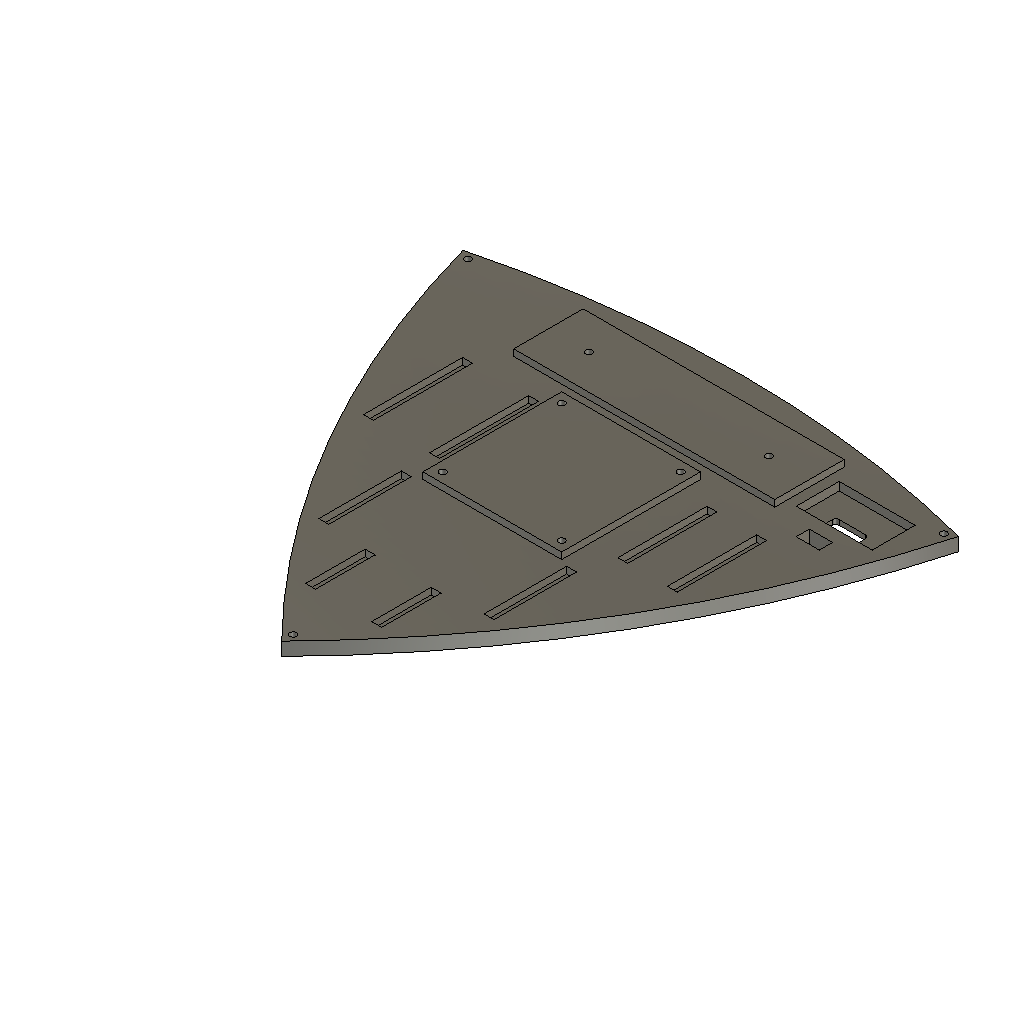
Body (Autodesk Fusion 360 design; units mm, degrees)
Autodesk Fusion 360 part; units mm, degrees
sketch "Base" plane through (0, 0, 0) normal (0, 0, 1) x (1, 0, 0)
  line L0 (0, 0) -> (150, 0)
  line L1 (150, 0) -> (75, -129.9038)
  line L2 (75, -129.9038) -> (0, 0)
  arc A0 (150, 0) -> (0, 0) centre (75, -290.4738) ccw
  arc A1 (0, 0) -> (75, -129.9038) centre (289.0576, 80.285) ccw
  arc A2 (75, -129.9038) -> (150, 0) centre (-139.0576, 80.285) ccw
  dimension "d1" = 150
  dimension "d2" = 150
  dimension "d3" = 150
  dimension "d4" = 300
  dimension "d5" = 300
  dimension "d6" = 300
  constraint coincident L0.start L2.end
  constraint horizontal L0
  measures "d1" distance of L0.start L0.end
  measures "d2" distance of L0.end L1.end
  measures "d3" distance of L0.start L1.end
  measures "d4" radius of A0
  measures "d5" radius of A1
  measures "d6" radius of A2
extrude "Extrude1" add sketch "Base" along normal blind 4
sketch "Pads" plane through (0, 0, 4) normal (0, 0, 1) x (-1, 0, 0)
  arc A0 (-75, 129.9038) -> (-150, 0) centre (139.0576, -80.285) ccw
  arc A1 (-150, 0) -> (0, 0) centre (-75, 290.4738) ccw
  arc A2 (0, 0) -> (-75, 129.9038) centre (-289.0576, -80.285) ccw
  line L0 (-54, 24.1538) -> (-96, 24.1538)
  line L1 (-96, 24.1538) -> (-96, 66.1538)
  line L2 (-96, 66.1538) -> (-54, 66.1538)
  line L3 (-54, 66.1538) -> (-54, 24.1538)
  line L4 (-114.5, 20.1538) -> (-35.5, 20.1538)
  line L5 (-35.5, 20.1538) -> (-35.5, -0.8462)
  line L6 (-35.5, -0.8462) -> (-114.5, -0.8462)
  line L7 (-114.5, -0.8462) -> (-114.5, 20.1538)
  dimension "d478" = 42
  dimension "d479" = 42
  dimension "d480" = 63.75
  dimension "d481" = 54
  dimension "d496" = 79
  dimension "d497" = 21
  dimension "d498" = 18.5
  dimension "d499" = 4
  constraint horizontal L0
  constraint vertical L1
  constraint horizontal L2
  constraint vertical L3
  constraint horizontal L4
  constraint vertical L5
  constraint horizontal L6
  constraint vertical L7
  measures "d478" distance of L0.start L0.end
  measures "d479" distance of L0.start L2.end
  measures "d480" distance of A0.start L2
  measures "d481" horizontal distance of A1.end L0.start
  measures "d496" distance of L4.start L4.end
  measures "d497" distance of L4.start L6.end
  measures "d498" distance of L3 L5
  measures "d499" distance of L0 L4
extrude "Extrude46" add sketch "Pads" along normal blind 2 contours L0 L1 L2 L3 | L4 L5 L6 L7
sketch "Clip holes" plane through (0, 0, 4) normal (0, 0, 1) x (-1, 0, 0)
  line L0 (-54, 24.1541) -> (-96, 24.1541)
  line L1 (-96, 24.1541) -> (-96, 66.1541)
  line L2 (-96, 66.1541) -> (-54, 66.1541)
  line L3 (-54, 66.1541) -> (-54, 24.1541)
  circle A0 centre (-3, 1.5) radius 0.75
  circle A1 centre (-147, 1.5) radius 0.75
  circle A2 centre (-75, 126.4038) radius 0.75
  arc A3 (-75, 129.9038) -> (-150, 0) centre (139.0576, -80.285) ccw
  arc A4 (-150, 0) -> (0, 0) centre (-75, 290.4738) ccw
  arc A5 (0, 0) -> (-75, 129.9038) centre (-289.0576, -80.285) ccw
  line L4 (-48.5, 92.1541) -> (-51.5, 92.1541)
  line L5 (-51.5, 92.1541) -> (-51.5, 67.1541)
  line L6 (-51.5, 67.1541) -> (-48.5, 67.1541)
  line L7 (-48.5, 67.1541) -> (-48.5, 92.1541)
  line L8 (-98.5, 92.1541) -> (-101.5, 92.1541)
  line L9 (-101.5, 92.1541) -> (-101.5, 67.1541)
  line L10 (-101.5, 67.1541) -> (-98.5, 67.1541)
  line L11 (-98.5, 67.1541) -> (-98.5, 92.1541)
  arc A6 (-75, 129.9038) -> (-150, 0) centre (139.0576, -80.285) ccw
  arc A7 (-150, 0) -> (0, 0) centre (-75, 290.4738) ccw
  arc A8 (0, 0) -> (-75, 129.9038) centre (-289.0576, -80.285) ccw
  line L12 (-66.5, 111.1541) -> (-63.5, 111.1541)
  line L13 (-63.5, 111.1541) -> (-63.5, 93.1541)
  line L14 (-63.5, 93.1541) -> (-66.5, 93.1541)
  line L15 (-66.5, 93.1541) -> (-66.5, 111.1541)
  line L16 (-83.5, 93.1541) -> (-86.5, 93.1541)
  line L17 (-86.5, 93.1541) -> (-86.5, 111.1541)
  line L18 (-86.5, 111.1541) -> (-83.5, 111.1541)
  line L19 (-83.5, 111.1541) -> (-83.5, 93.1541)
  line L20 (-28, 58.1538) -> (-28, 28.1538)
  line L21 (-28, 28.1538) -> (-31, 28.1538)
  line L22 (-31, 58.1538) -> (-28, 58.1538)
  line L23 (-31, 28.1538) -> (-31, 58.1538)
  line L24 (-54, 66.1538) -> (-54, 24.1538)
  line L25 (-54, 24.1538) -> (-96, 24.1538)
  line L26 (-96, 24.1538) -> (-96, 66.1538)
  line L27 (-96, 66.1538) -> (-54, 66.1538)
  line L28 (-114.5, -0.8462) -> (-114.5, 20.1538)
  line L29 (-114.5, 20.1538) -> (-35.5, 20.1538)
  line L30 (-35.5, 20.1538) -> (-35.5, -0.8462)
  line L31 (-35.5, -0.8462) -> (-114.5, -0.8462)
  line L32 (-104, 30.1538) -> (-107, 30.1538)
  line L33 (-107, 30.1538) -> (-107, 57.1538)
  line L34 (-107, 57.1538) -> (-104, 57.1538)
  line L35 (-104, 57.1538) -> (-104, 30.1538)
  line L36 (-119, 30.1538) -> (-122, 30.1538)
  line L37 (-122, 30.1538) -> (-122, 57.1538)
  line L38 (-122, 57.1538) -> (-119, 57.1538)
  line L39 (-119, 57.1538) -> (-119, 30.1538)
  line L40 (-48, 28.1538) -> (-51, 28.1538)
  line L41 (-51, 28.1538) -> (-51, 58.1538)
  line L42 (-51, 58.1538) -> (-48, 58.1538)
  line L43 (-48, 58.1538) -> (-48, 28.1538)
  line L44 (-96, 24.1538) -> (-54, 24.1538)
  dimension "d427" = 25
  dimension "d428" = 25
  dimension "d468" = 18
  dimension "d469" = 3
  dimension "d471" = 3
  dimension "d472" = 18
  dimension "d474" = 30
  dimension "d475" = 3
  dimension "d559" = 3
  dimension "d560" = 3
  dimension "d561" = 3
  dimension "d562" = 27
  dimension "d563" = 10
  dimension "d564" = 3
  dimension "d565" = 27
  dimension "d566" = 10
  dimension "d567" = 18
  dimension "d568" = 8
  dimension "d569" = 23
  dimension "d570" = 1
  dimension "d571" = 1
  dimension "d572" = 1
  dimension "d573" = 53
  dimension "d574" = 2.5
  dimension "d575" = 1
  dimension "d579" = 3
  dimension "d580" = 30
  dimension "d581" = 23
  dimension "d583" = 4
  dimension "d584" = 4
  dimension "d585" = 3
  dimension "d586" = 12
  constraint horizontal L4
  constraint vertical L5
  constraint horizontal L6
  constraint vertical L7
  constraint horizontal L8
  constraint vertical L9
  constraint horizontal L10
  constraint vertical L11
  constraint horizontal L12
  constraint vertical L13
  constraint horizontal L14
  constraint vertical L15
  constraint horizontal L16
  constraint vertical L17
  constraint horizontal L18
  constraint vertical L19
  constraint horizontal L22
  constraint vertical L20
  constraint horizontal L21
  constraint vertical L23
  constraint horizontal L32
  constraint vertical L33
  constraint horizontal L34
  constraint vertical L35
  constraint horizontal L36
  constraint vertical L37
  constraint horizontal L38
  constraint vertical L39
  constraint horizontal L40
  constraint vertical L41
  constraint horizontal L42
  constraint vertical L43
  measures "d427" distance of L4.start L6.end
  measures "d428" distance of L8.end L9.end
  measures "d468" distance of L12.start L14.end
  measures "d469" distance of L13.end L14.end
  measures "d471" distance of L16.start L16.end
  measures "d472" distance of L16.start L18.end
  measures "d474" distance of L21.end L22.start
  measures "d475" distance of L21.end L20.end
  measures "d559" distance of L5 L7
  measures "d560" distance of L9 L11
  measures "d561" distance of L32.start L32.end
  measures "d562" distance of L32.start L34.end
  measures "d563" distance of L29 L32
  measures "d564" distance of L36.start L36.end
  measures "d565" distance of L36.start L38.end
  measures "d566" distance of L29 L36
  measures "d567" distance of L35 L37
  measures "d568" distance of L1 L35
  measures "d569" distance of L13 L17
  measures "d570" distance of L4 L14
  measures "d571" distance of L8 L16
  measures "d572" distance of L2 L6
  measures "d573" distance of L7 L9
  measures "d574" distance of L3 L5
  measures "d575" distance of L2 L10
  measures "d579" distance of L40.start L40.end
  measures "d580" distance of L40.start L42.end
  measures "d581" distance of L20 L41
  measures "d583" distance of L40 L44
  measures "d584" distance of L21 L44
  measures "d585" distance of L3 L41
  measures "d586" distance of L5 L13
extrude "Extrude39" cut sketch "Clip holes" against normal blind 2 contours L4 L5 L6 L7 | L8 L9 L10 L11 | L12 L13 L14 L15 | L16 L17 L18 L19 | L20 L21 L22 L23 | L32 L33 L34 L35 | L36 L37 L38 L39 | L40 L41 L42 L43
sketch "Charger" plane through (0, 0, 4) normal (0, 0, 1) x (-1, 0, 0)
  arc A0 (-75, 129.9038) -> (-150, 0) centre (139.0576, -80.285) ccw
  arc A1 (-150, 0) -> (0, 0) centre (-75, 290.4738) ccw
  arc A2 (0, 0) -> (-75, 129.9038) centre (-289.0576, -80.285) ccw
  line L0 (-54, 24.1538) -> (-96, 24.1538)
  line L1 (-96, 24.1538) -> (-96, 66.1538)
  line L2 (-96, 66.1538) -> (-54, 66.1538)
  line L3 (-54, 66.1538) -> (-54, 24.1538)
  line L4 (-114.5, -0.8462) -> (-114.5, 20.1538)
  line L5 (-114.5, 20.1538) -> (-35.5, 20.1538)
  line L6 (-35.5, 20.1538) -> (-35.5, -0.8462)
  line L7 (-35.5, -0.8462) -> (-114.5, -0.8462)
  line L8 (-86.5, 93.1541) -> (-86.5, 111.1541)
  line L9 (-86.5, 111.1541) -> (-83.5, 111.1541)
  line L10 (-83.5, 111.1541) -> (-83.5, 93.1541)
  line L11 (-83.5, 93.1541) -> (-86.5, 93.1541)
  line L12 (-51.5, 92.1541) -> (-48.5, 92.1541)
  line L13 (-48.5, 92.1541) -> (-48.5, 67.1541)
  line L14 (-48.5, 67.1541) -> (-51.5, 67.1541)
  line L15 (-51.5, 67.1541) -> (-51.5, 92.1541)
  line L16 (-28, 58.1538) -> (-28, 28.1538)
  line L17 (-28, 28.1538) -> (-31, 28.1538)
  line L18 (-31, 28.1538) -> (-31, 58.1538)
  line L19 (-31, 58.1538) -> (-28, 58.1538)
  line L20 (-63.5, 111.1541) -> (-63.5, 93.1541)
  line L21 (-63.5, 93.1541) -> (-66.5, 93.1541)
  line L22 (-66.5, 93.1541) -> (-66.5, 111.1541)
  line L23 (-66.5, 111.1541) -> (-63.5, 111.1541)
  line L24 (-101.5, 92.1541) -> (-98.5, 92.1541)
  line L25 (-98.5, 92.1541) -> (-98.5, 67.1541)
  line L26 (-98.5, 67.1541) -> (-101.5, 67.1541)
  line L27 (-101.5, 67.1541) -> (-101.5, 92.1541)
  line L28 (-117.5, 3.6538) -> (-140.5, 3.6538)
  line L29 (-140.5, 3.6538) -> (-140.5, 16.6538)
  line L30 (-140.5, 16.6538) -> (-117.5, 16.6538)
  line L31 (-117.5, 16.6538) -> (-117.5, 3.6538)
  line L32 (-122, 30.1538) -> (-122, 57.1538)
  line L33 (-122, 57.1538) -> (-119, 57.1538)
  line L34 (-119, 57.1538) -> (-119, 30.1538)
  line L35 (-119, 30.1538) -> (-122, 30.1538)
  line L36 (-107, 30.1538) -> (-107, 57.1538)
  line L37 (-107, 57.1538) -> (-104, 57.1538)
  line L38 (-104, 57.1538) -> (-104, 30.1538)
  line L39 (-104, 30.1538) -> (-107, 30.1538)
  line L40 (-51, 28.1538) -> (-51, 58.1538)
  line L41 (-51, 58.1538) -> (-48, 58.1538)
  line L42 (-48, 58.1538) -> (-48, 28.1538)
  line L43 (-48, 28.1538) -> (-51, 28.1538)
  dimension "d539" = 23
  dimension "d540" = 13
  dimension "d541" = 3
  dimension "d542" = 4.5
  constraint horizontal L28
  constraint vertical L29
  constraint horizontal L30
  constraint vertical L31
  measures "d539" distance of L28.start L28.end
  measures "d540" distance of L28.start L30.end
  measures "d541" distance of L4 L31
  measures "d542" distance of L7 L28
extrude "Extrude56" cut sketch "Charger" against normal blind 2.5 contours L28 L29 L30 L31
sketch "Switch" plane through (0, 0, 4) normal (0, 0, 1) x (-1, 0, 0)
  line L0 (-101.5, 92.1541) -> (-98.5, 92.1541)
  line L1 (-98.5, 92.1541) -> (-98.5, 67.1541)
  line L2 (-98.5, 67.1541) -> (-101.5, 67.1541)
  line L3 (-101.5, 67.1541) -> (-101.5, 92.1541)
  line L4 (-63.5, 111.1541) -> (-63.5, 93.1541)
  line L5 (-63.5, 93.1541) -> (-66.5, 93.1541)
  line L6 (-66.5, 93.1541) -> (-66.5, 111.1541)
  line L7 (-66.5, 111.1541) -> (-63.5, 111.1541)
  line L8 (-28, 58.1538) -> (-28, 28.1538)
  line L9 (-28, 28.1538) -> (-31, 28.1538)
  line L10 (-31, 28.1538) -> (-31, 58.1538)
  line L11 (-31, 58.1538) -> (-28, 58.1538)
  line L12 (-51.5, 92.1541) -> (-48.5, 92.1541)
  line L13 (-48.5, 92.1541) -> (-48.5, 67.1541)
  line L14 (-48.5, 67.1541) -> (-51.5, 67.1541)
  line L15 (-51.5, 67.1541) -> (-51.5, 92.1541)
  line L16 (-86.5, 93.1541) -> (-86.5, 111.1541)
  line L17 (-86.5, 111.1541) -> (-83.5, 111.1541)
  line L18 (-83.5, 111.1541) -> (-83.5, 93.1541)
  line L19 (-83.5, 93.1541) -> (-86.5, 93.1541)
  line L20 (-114.5, -0.8462) -> (-114.5, 20.1538)
  line L21 (-114.5, 20.1538) -> (-35.5, 20.1538)
  line L22 (-35.5, 20.1538) -> (-35.5, -0.8462)
  line L23 (-35.5, -0.8462) -> (-114.5, -0.8462)
  line L24 (-54, 24.1538) -> (-96, 24.1538)
  line L25 (-96, 24.1538) -> (-96, 66.1538)
  line L26 (-96, 66.1538) -> (-54, 66.1538)
  line L27 (-54, 66.1538) -> (-54, 24.1538)
  arc A0 (-75, 129.9038) -> (-150, 0) centre (139.0576, -80.285) ccw
  arc A1 (-150, 0) -> (0, 0) centre (-75, 290.4738) ccw
  arc A2 (0, 0) -> (-75, 129.9038) centre (-289.0576, -80.285) ccw
  line L28 (-140.5, 3.6538) -> (-140.5, 16.6538)
  line L29 (-140.5, 16.6538) -> (-117.5, 16.6538)
  line L30 (-117.5, 16.6538) -> (-117.5, 3.6538)
  line L31 (-117.5, 3.6538) -> (-140.5, 3.6538)
  line L32 (-125.5, 20.6538) -> (-132.5, 20.6538)
  line L33 (-132.5, 20.6538) -> (-132.5, 24.6538)
  line L34 (-132.5, 24.6538) -> (-125.5, 24.6538)
  line L35 (-125.5, 24.6538) -> (-125.5, 20.6538)
  line L36 (-107, 30.1538) -> (-107, 57.1538)
  line L37 (-107, 57.1538) -> (-104, 57.1538)
  line L38 (-104, 57.1538) -> (-104, 30.1538)
  line L39 (-104, 30.1538) -> (-107, 30.1538)
  line L40 (-122, 30.1538) -> (-122, 57.1538)
  line L41 (-122, 57.1538) -> (-119, 57.1538)
  line L42 (-119, 57.1538) -> (-119, 30.1538)
  line L43 (-119, 30.1538) -> (-122, 30.1538)
  line L44 (-51, 28.1538) -> (-51, 58.1538)
  line L45 (-51, 58.1538) -> (-48, 58.1538)
  line L46 (-48, 58.1538) -> (-48, 28.1538)
  line L47 (-48, 28.1538) -> (-51, 28.1538)
  dimension "d545" = 7
  dimension "d546" = 4
  dimension "d547" = 4
  dimension "d548" = 8
  constraint horizontal L32
  constraint vertical L33
  constraint horizontal L34
  constraint vertical L35
  measures "d545" distance of L32.start L32.end
  measures "d546" distance of L32.start L34.end
  measures "d547" distance of L29 L32
  measures "d548" distance of L30 L35
extrude "Extrude57" cut sketch "Switch" against normal blind 4 contours L32 L33 L34 L35
sketch "Charger hole" plane through (0, 0, 1.5) normal (0, 0, 1) x (-1, 0, 0)
  line L0 (-117.5, 16.6538) -> (-140.5, 16.6538)
  line L1 (-140.5, 16.6538) -> (-140.5, 3.6538)
  line L2 (-140.5, 3.6538) -> (-117.5, 3.6538)
  line L3 (-117.5, 3.6538) -> (-117.5, 16.6538)
  line L4 (-124, 11.1538) -> (-134, 11.1538)
  line L5 (-134, 11.1538) -> (-134, 15.1538)
  line L6 (-134, 15.1538) -> (-124, 15.1538)
  line L7 (-124, 15.1538) -> (-124, 11.1538)
  dimension "d551" = 10
  dimension "d552" = 4
  dimension "d554" = 6.5
  dimension "d617" = 1.5
  constraint horizontal L4
  constraint vertical L5
  constraint horizontal L6
  constraint vertical L7
  measures "d551" distance of L4.start L4.end
  measures "d552" distance of L4.start L6.end
  measures "d554" distance of L3 L7
  measures "d617" distance of L0 L6
extrude "Extrude58" cut sketch "Charger hole" against normal blind 1.5 contours L4 L5 L6 L7
fillet "Fillet10" radius 1 4 edges at (124, -11.1538, 0.75) (124, -15.1538, 0.75) (134, -15.1538, 0.75) (134, -11.1538, 0.75)
sketch "Motor holes" plane through (0, 0, 6) normal (0, 0, 1) x (-1, 0, 0)
  line L0 (-54, 66.1538) -> (-96, 66.1538)
  line L1 (-96, 66.1538) -> (-96, 24.1538)
  line L2 (-96, 24.1538) -> (-54, 24.1538)
  line L3 (-54, 24.1538) -> (-54, 66.1538)
  circle A0 centre (-57, 27.1538) radius 1
  circle A1 centre (-93, 27.1538) radius 1
  circle A2 centre (-93, 63.1538) radius 1
  circle A3 centre (-57, 63.1538) radius 1
  dimension "d587" = 2
  dimension "d588" = 3
  dimension "d589" = 3
  dimension "d590" = 2
  dimension "d591" = 3
  dimension "d592" = 3
  dimension "d593" = 2
  dimension "d594" = 3
  dimension "d595" = 3
  dimension "d596" = 2
  dimension "d597" = 3
  dimension "d598" = 3
  measures "d587" diameter of A0
  measures "d588" distance of L2 A0.centre
  measures "d589" distance of L3 A0.centre
  measures "d590" diameter of A1
  measures "d591" distance of L2 A1.centre
  measures "d592" distance of L1 A1.centre
  measures "d593" diameter of A2
  measures "d594" distance of L1 A2.centre
  measures "d595" distance of L0 A2.centre
  measures "d596" diameter of A3
  measures "d597" distance of L3 A3.centre
  measures "d598" distance of L0 A3.centre
sketch "Battery holes" plane through (0, 0, 6) normal (0, 0, 1) x (-1, 0, 0)
  line L0 (-114.5, -0.8462) -> (-35.5, -0.8462)
  line L1 (-35.5, -0.8462) -> (-35.5, 20.1538)
  line L2 (-35.5, 20.1538) -> (-114.5, 20.1538)
  line L3 (-114.5, 20.1538) -> (-114.5, -0.8462)
  circle A0 centre (-47.75, 9.6538) radius 1
  circle A1 centre (-102.25, 9.6538) radius 1
  dimension "d599" = 2
  dimension "d600" = 2
  dimension "d601" = 10.5
  dimension "d602" = 10.5
  dimension "d603" = 54.5
  dimension "d604" = 12.25
  measures "d599" diameter of A0
  measures "d600" diameter of A1
  measures "d601" distance of L0 A0.centre
  measures "d602" distance of L0 A1.centre
  measures "d603" distance of A0.centre A1.centre
  measures "d604" distance of L1 A0.centre
extrude "Extrude59" cut sketch "Battery holes" sketch "Motor holes" against normal blind 4 contours A0 | A1 of sketch 2 contours A0 | A1 | A2 | A3
sketch "Case holes" plane through (0, 0, 4) normal (0, 0, 1) x (-1, 0, 0)
  line L0 (-140.5, 3.6538) -> (-140.5, 16.6538)
  line L1 (-140.5, 16.6538) -> (-117.5, 16.6538)
  line L2 (-117.5, 16.6538) -> (-117.5, 3.6538)
  line L3 (-117.5, 3.6538) -> (-140.5, 3.6538)
  arc A0 (-75, 129.9038) -> (-150, 0) centre (139.0576, -80.285) ccw
  arc A1 (-150, 0) -> (0, 0) centre (-75, 290.4738) ccw
  arc A2 (0, 0) -> (-75, 129.9038) centre (-289.0576, -80.285) ccw
  line L4 (-54, 66.1538) -> (-54, 24.1538)
  line L5 (-54, 24.1538) -> (-96, 24.1538)
  line L6 (-96, 24.1538) -> (-96, 66.1538)
  line L7 (-96, 66.1538) -> (-54, 66.1538)
  line L8 (-114.5, -0.8462) -> (-114.5, 20.1538)
  line L9 (-114.5, 20.1538) -> (-35.5, 20.1538)
  line L10 (-35.5, 20.1538) -> (-35.5, -0.8462)
  line L11 (-35.5, -0.8462) -> (-114.5, -0.8462)
  line L12 (-51, 28.1538) -> (-51, 58.1538)
  line L13 (-51, 58.1538) -> (-48, 58.1538)
  line L14 (-48, 58.1538) -> (-48, 28.1538)
  line L15 (-48, 28.1538) -> (-51, 28.1538)
  line L16 (-63.5, 111.1541) -> (-63.5, 93.1541)
  line L17 (-63.5, 93.1541) -> (-66.5, 93.1541)
  line L18 (-66.5, 93.1541) -> (-66.5, 111.1541)
  line L19 (-66.5, 111.1541) -> (-63.5, 111.1541)
  line L20 (-101.5, 92.1541) -> (-98.5, 92.1541)
  line L21 (-98.5, 92.1541) -> (-98.5, 67.1541)
  line L22 (-98.5, 67.1541) -> (-101.5, 67.1541)
  line L23 (-101.5, 67.1541) -> (-101.5, 92.1541)
  line L24 (-86.5, 93.1541) -> (-86.5, 111.1541)
  line L25 (-86.5, 111.1541) -> (-83.5, 111.1541)
  line L26 (-83.5, 111.1541) -> (-83.5, 93.1541)
  line L27 (-83.5, 93.1541) -> (-86.5, 93.1541)
  line L28 (-122, 30.1538) -> (-122, 57.1538)
  line L29 (-122, 57.1538) -> (-119, 57.1538)
  line L30 (-119, 57.1538) -> (-119, 30.1538)
  line L31 (-119, 30.1538) -> (-122, 30.1538)
  line L32 (-28, 58.1538) -> (-28, 28.1538)
  line L33 (-28, 28.1538) -> (-31, 28.1538)
  line L34 (-31, 28.1538) -> (-31, 58.1538)
  line L35 (-31, 58.1538) -> (-28, 58.1538)
  line L36 (-51.5, 92.1541) -> (-48.5, 92.1541)
  line L37 (-48.5, 92.1541) -> (-48.5, 67.1541)
  line L38 (-48.5, 67.1541) -> (-51.5, 67.1541)
  line L39 (-51.5, 67.1541) -> (-51.5, 92.1541)
  line L40 (-107, 30.1538) -> (-107, 57.1538)
  line L41 (-107, 57.1538) -> (-104, 57.1538)
  line L42 (-104, 57.1538) -> (-104, 30.1538)
  line L43 (-104, 30.1538) -> (-107, 30.1538)
  line L44 (-132.5, 20.6538) -> (-132.5, 24.6538)
  line L45 (-132.5, 24.6538) -> (-125.5, 24.6538)
  line L46 (-125.5, 24.6538) -> (-125.5, 20.6538)
  line L47 (-125.5, 20.6538) -> (-132.5, 20.6538)
  circle A3 centre (-75.0001, 126.4038) radius 1
  circle A4 centre (-3, 1.5) radius 1
  circle A5 centre (-147, 1.5) radius 1
  dimension "d607" = 2
  dimension "d608" = 2
  dimension "d609" = 3
  dimension "d610" = 1.5
  dimension "d611" = 2
  dimension "d612" = 3
  dimension "d613" = 1.5
  dimension "d614" = 3.5
  measures "d607" diameter of A3
  measures "d608" diameter of A4
  measures "d609" horizontal distance of A1.end A4.centre
  measures "d610" vertical distance of A1.end A4.centre
  measures "d611" diameter of A5
  measures "d612" horizontal distance of A0.end A5.centre
  measures "d613" vertical distance of A0.end A5.centre
  measures "d614" vertical distance of A0.start A3.centre
extrude "Extrude60" cut sketch "Case holes" against normal blind 4 contours A3 | A4 | A5
equation "CLIP_PCB_SIZE = 16 mm"
equation "CLIP_PCB_THICKNESS = 1 mm"
equation "CLIP_DISTANCE_TO_BASE = 7 mm"
equation "CLIP_THICKNESS = 4 mm"
